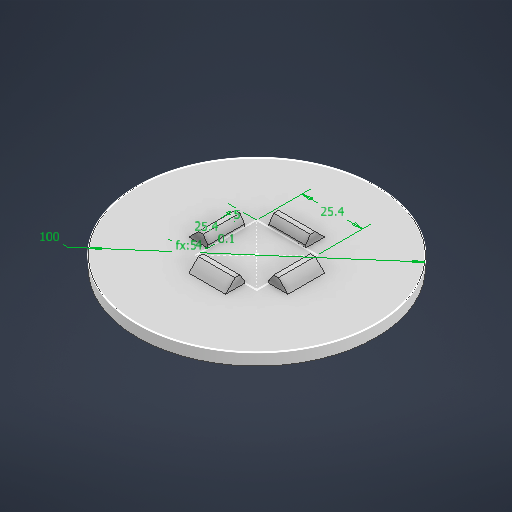
# Autodesk Inventor part: Spin Chuck
Saved by Autodesk Inventor 2025.1 (Build 291241000, 241)
## iProperties
Created: 2024-11-11
Part Number: Spin Chuck
Material: Generic
Document SubType Name: Modeling
Designer: jerem
Density: 1 g/cm^3
Appearance: Default
Author: jerem
Autodesk Inventor part; units mm, degrees
ref_plane "YZ Plane" through (0, 0, 0) normal (1, 0, 0) x (0, 1, 0)
ref_plane "XZ Plane" through (0, 0, 0) normal (0, 1, 0) x (-1, 0, 0)
ref_plane "XY Plane" through (0, 0, 0) normal (0, 0, 1) x (1, 0, 0)
sketch "Sketch1" plane through (0, 0, 0) normal (0, 1, 0) x (-1, 0, 0)
  line L0 (-12.7, 12.7) -> (12.7, 12.7)
  line L1 (12.7, 12.7) -> (12.7, -12.7)
  line L2 (12.7, -12.7) -> (-12.7, -12.7)
  line L3 (-12.7, -12.7) -> (-12.7, 12.7)
  line L4 (-12.7, 12.7) -> (12.7, -12.7) construction
  line L5 (12.7, 12.7) -> (-12.7, -12.7) construction
  circle A0 centre (0, 0) radius 50
  line L6 (12.8, -7.7) -> (16.8, -7.7)
  line L7 (16.8, -7.7) -> (16.8, 7.7)
  line L8 (16.8, 7.7) -> (12.8, 7.7)
  line L9 (12.8, 7.7) -> (12.8, -7.7)
  dimension "d0" = 25.4
  dimension "d1" = 25.4
  dimension "d2" = 0.1
  dimension "d3" = 4
  dimension "d4" = 100
  dimension "d7" = 5
  dimension "d8" = 5
  constraints: 20 end point, 4 parallel, 2 horizontal, 2 midpoint, 2 perpendicular, 1 centre point, 1 coincident
  measures "d0" distance of L1.end L2.end
  measures "d1" distance of L0.end L1.end
  measures "d2" distance between parallel lines of L1 L9
  measures "d3" distance of L7.end L8.end
  measures "d4" diameter of A0
  measures "d7" distance between parallel lines of L2 L6
  measures "d8" distance between parallel lines of L0 L8
extrude "Extrusion1" add sketch "Sketch1" against normal blind 5 contours L0 L1 L2 L3 | A0 | L9 L8 L7 L6
extrude "Extrusion2" add sketch "Sketch1" along normal blind 4 contours L9 L8 L7 L6
chamfer "Chamfer1" distance 2 distance2 3 1 edges at (-12.8, 4, 0) measured on face at (-13.3, 4, 0)
chamfer "Chamfer2" distance 4 angle 45 1 edges at (-16.8, 0, 0)
pattern_circular "Circular Pattern1" count 4 over 360 about axis through (0, 0, 0) along (0, -1, 0) of "Extrusion2", "Chamfer2", "Chamfer1"
equation "\"d8\" = d7"
body "Solid1"
